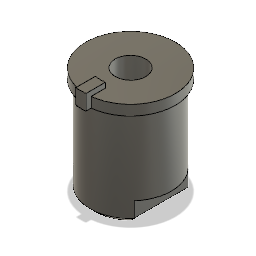
PinionGearExt (Autodesk Fusion 360 design; units mm, degrees)
Autodesk Fusion 360 part; units mm, degrees
sketch "Sketch1" plane through (0, 0, 0) normal (0, 1, 0) x (1, 0, 0)
  circle A0 centre (0, 0) radius 4
  dimension "d1" = 8
  constraint coincident A0.centre origin
  measures "d1" diameter of A0
extrude "Extrude1" add sketch "Sketch1" along normal blind 7.5
sketch "Sketch2" plane through (0, 7.5, 0) normal (0, 1, 0) x (-1, 0, 0)
  circle A0 centre (0, 0) radius 4
  circle A1 centre (0, 0) radius 4.4
  dimension "d4" = 0.4
  constraint concentric A0 A1
  measures "d4" distance of A0 A1
extrude "Extrude2" add sketch "Sketch2" along normal blind 1 contours A0 | A1
sketch "Sketch3" plane through (0, 0, 0) normal (0, -1, 0) x (1, 0, 0)
  circle A0 centre (0, 0) radius 4
  line L0 (-3, 2.6458) -> (-3, -2.6458)
  line L1 (-3, -2.6458) -> (0, -4)
  line L2 (0, -4) -> (3, -2.6458)
  line L3 (3, -2.6458) -> (3, 2.6458)
  line L4 (-3, 0) -> (3, 0) construction
  dimension "d7" = 6
  constraint coincident A0 L0.start
  constraint coincident A0 L0.end
  constraint coincident A0 L1.end
  constraint coincident A0 L2.end
  constraint coincident A0 L3.end
  constraint vertical L3
  constraint vertical L0
  constraint equal L1 L2
  constraint midpoint L0 L4.start
  constraint midpoint L3 L4.end
  constraint midpoint A0.centre L4
  measures "d7" distance of L4.start L4.end
extrude "Extrude3" add sketch "Sketch3" along normal blind 2 contours A0 L0 L1 L2 L3
sketch "Sketch4" plane through (0, -2, 0) normal (0, -1, 0) x (1, 0, 0)
  line L0 (3, -2.6458) -> (3, 2.6458)
  arc A0 (3, 2.6458) -> (-3, 2.6458) centre (0, 0) ccw
  line L1 (-3, 2.6458) -> (-3, -2.6458)
  line L2 (-3, -2.6458) -> (0, -4)
  line L3 (0, -4) -> (3, -2.6458)
  circle A1 centre (0, 0) radius 1.5
  dimension "d10" = 3
  constraint concentric A0 A1
  measures "d10" diameter of A1
extrude "Extrude4" cut sketch "Sketch4" against normal through all contours A1
chamfer "Chamfer1" distance 0.5 angle 45 5 edges at (0, -2, 4) (-3, -2, 0) (-1.5, -2, -3.3229) (1.5, -2, -3.3229) (3, -2, 0)
sketch "Sketch5" plane through (0, 8.5, 0) normal (0, 1, 0) x (-1, 0, 0)
  circle A0 centre (0, 0) radius 1.5
  circle A1 centre (0, 0) radius 4.4
  circle A2 centre (0, 0) radius 3
  line L0 (0, 0) -> (0, 5.5) construction
  line L1 (-0.5, 2.958) -> (-0.5, 4.3715)
  line L2 (0.5, 2.958) -> (0.5, 4.3715)
  dimension "d13" = 6
  dimension "d17" = 1
  constraint concentric A0 A2
  constraint coincident A0.centre A1.centre
  constraint vertical L0
  constraint coincident A2 L1.start
  constraint coincident A1 L1.end
  constraint vertical L1
  constraint symmetric L0 L1.start L2.start
  constraint symmetric L0 L1.end L2.end
  measures "d13" diameter of A2
  measures "d17" distance of L1.start L2.start
extrude "Extrude5" add sketch "Sketch5" along normal blind 0.5 contours A1 A2 L1 L2 picked at (0.3891, 3.4416)
sketch "Sketch7" plane through (0, 9, 0) normal (0, 1, 0) x (-1, 0, 0)
  arc A0 (0.5, 2.958) -> (-0.5, 2.958) centre (0, 0) ccw
  line L0 (0.5, 2.958) -> (0.5, 4.3715)
  arc A1 (0.5, 4.3715) -> (-0.5, 4.3715) centre (0, 0) ccw
  line L1 (-0.5, 4.3715) -> (-0.5, 2.958)
  arc A2 (-0.5, 4.3715) -> (0.5, 4.3715) centre (0, 0) ccw
  line L2 (0.5, 4.3715) -> (0.5, 4.8744)
  line L3 (-0.5, 4.3715) -> (-0.5, 4.8744)
  arc A3 (0.5, 4.8744) -> (-0.5, 4.8744) centre (0, 0) ccw
  dimension "d18" = 0.5
  constraint concentric A0 A3
  constraint coincident L0.end A1.start
  constraint vertical L2
  constraint coincident A1.end L1.start
  constraint parallel L1 L3
  measures "d18" distance of A2 A3
extrude "Extrude6" add sketch "Sketch7" against normal blind 1.5 contours A1 L2 L3 A3
equation "d2 = ( 2 * 3.25 ) * 1 mm + 1 mm"
